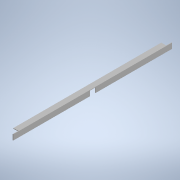
# Autodesk Inventor part: A_3030_INT
Saved by Autodesk Inventor 2020 (Build 240168000, 168)
## iProperties
Created: 2022-04-18
Part Number: A_3030_INT
Material: Genérico
Document SubType Name: Modeling
Designer: aarco
Density: 1 g/cm^3
Appearance: Valor por defecto
Author: aarco
Autodesk Inventor part; units mm, degrees
ref_plane "YZ Plane" through (0, 0, 0) normal (1, 0, 0) x (0, 1, 0)
ref_plane "XZ Plane" through (0, 0, 0) normal (0, 1, 0) x (-1, 0, 0)
ref_plane "XY Plane" through (0, 0, 0) normal (0, 0, 1) x (1, 0, 0)
sketch "Boceto1" plane through (0, 0, 0) normal (0, 1, 0) x (-1, 0, 0)
  line L0 (27, 411.5) -> (0, 411.5)
  line L1 (0, 411.5) -> (0, -411.5)
  line L2 (0, -411.5) -> (27, -411.5)
  line L3 (27, -411.5) -> (27, 411.5)
  line L4 (0, 0) -> (280.3389, 0)
  dimension "d0" = 823
  dimension "d1" = 27
  constraints: 10 end point, 2 horizontal, 2 parallel, 1 midpoint, 1 perpendicular, 1 symmetric about line
  measures "d0" distance of L2.end L0.start
  measures "d1" distance of L0.start L0.end
extrude "Extrusión1" add sketch "Boceto1" along normal blind 3
sketch "Boceto2" plane through (0, 3, 0) normal (0, 1, 0) x (1, 0, 0)
  line L0 (0, -441.5) -> (3, -441.5)
  line L1 (3, -441.5) -> (3, 441.5)
  line L2 (3, 441.5) -> (0, 441.5)
  line L3 (0, 441.5) -> (0, -441.5)
  line L4 (0, 0) -> (-318.7817, 0)
  point P0 (0, -411.5)
  dimension "d4" = 883
  dimension "d5" = 3
  constraints: 10 end point, 2 horizontal, 2 parallel, 1 perpendicular, 1 point on line, 1 symmetric about line
  measures "d4" distance of L0.end L1.end
  measures "d5" distance of L0.start L0.end
extrude "Extrusión2" add sketch "Boceto2" against normal blind 30
sketch "Boceto3" plane through (3, 3, 441.5) normal (1, 0, 0) x (0, 0, -1)
  line L0 (883, -30) -> (0, -30) projected
  line L1 (441.5, -30) -> (441.5, 0)
  line L2 (853, 0) -> (30, 0) projected
  line L3 (456.5, -30) -> (426.5, -30)
  line L4 (426.5, -30) -> (426.5, 0)
  line L5 (426.5, 0) -> (456.5, 0)
  line L6 (456.5, 0) -> (456.5, -30)
  line L7 (0, 0) -> (883, 0) projected
  line L8 (30, -3) -> (853, -3) projected
  point P0 (441.5, -3)
  point P1 (456.5, -3)
  point P2 (426.5, -3)
  dimension "d8" = 30
  constraints: 10 end point, 6 midpoint, 2 parallel, 1 horizontal, 1 perpendicular, 1 point on line
  measures "d8" distance between parallel lines of L4 L6
extrude "Extrusión3" cut sketch "Boceto3" against normal blind 10 contours L0 L1 L8 L6 | L0 L4 L8 L1
fillet "Empalme1" radius 2 2 edges at (1.5, -27, 15) (1.5, -27, -15)
